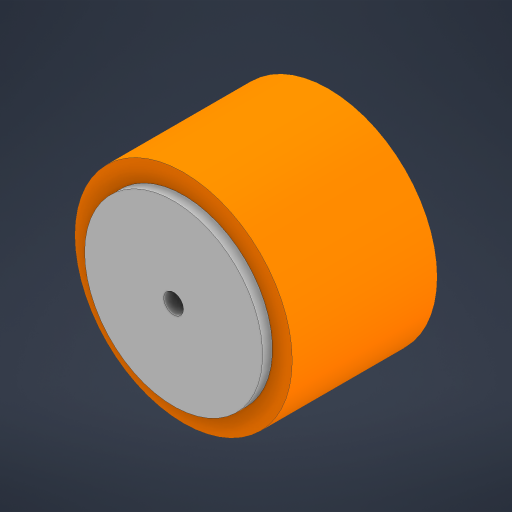
# Autodesk Inventor part: JSUMO_Wheel_33x20mm
Saved by Autodesk Inventor 2024 (Build 280153000, 153)
## iProperties
Created: 2024-01-29
Part Number: JSUMO_Wheel_33x20mm
Material: Všeobecné
Document SubType Name: Modeling
Designer: 42060
Density: 1 g/cm^3
Appearance: Výchozí
Author: 42060
Autodesk Inventor part; units mm, degrees
ref_plane "YZ Plane" through (0, 0, 0) normal (1, 0, 0) x (0, 1, 0)
ref_plane "XZ Plane" through (0, 0, 0) normal (0, 1, 0) x (-1, 0, 0)
ref_plane "XY Plane" through (0, 0, 0) normal (0, 0, 1) x (1, 0, 0)
sketch "Náčrt1" plane through (0, 0, 0) normal (0, 1, 0) x (-1, 0, 0)
  circle A0 centre (0, 0) radius 16.5
  circle A1 centre (0, 0) radius 13.5
  dimension "d0" = 33
  dimension "d1" = 27
  constraints: 2 centre point, 2 coincident
  measures "d0" diameter of A0
  measures "d1" diameter of A1
extrude "Vysunutí1" add sketch "Náčrt1" along normal mid plane 25 contours A1
sketch "Náčrt4" plane through (0, 0, 0) normal (1, 0, 0) x (0, 1, 0)
  line L0 (-12.5, 13.5) -> (-12.5, -13.5) projected
  point P0 (0, 0)
  point P1 (-8.5, 0)
  dimension "d16" = 4
  measures "d16" distance from line of L0 point (-8.5, 0)
hole "Díra2" at (0, -8.5, 0) direction (1, 0, 0) diameter 3 end through all
thread "Závit1" size "M3x0.5" class "6H" standard "ISO Metric profile" full length
extrude "Vysunutí2" add sketch "Náčrt1" along normal mid plane 22
sketch "Náčrt2" plane through (0, 12.5, 0) normal (0, 1, 0) x (1, 0, 0)
  circle A0 centre (0, 0) radius 9
  dimension "d6" = 18
  constraints: 1 centre point, 1 coincident
  measures "d6" diameter of A0
extrude "Vysunutí3" cut sketch "Náčrt2" against normal blind 14.5
sketch "Náčrt3" plane through (0, -12.5, 0) normal (0, -1, 0) x (1, 0, 0)
  circle A0 centre (0, 0) radius 13.5 projected
  constraints: 1 coincident
hole "Díra1" at (0, -12.5, 0) direction (0, 1, 0) diameter 3 end through all
